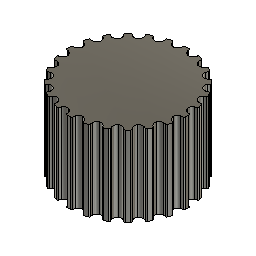
gear_24z (Autodesk Fusion 360 design; units mm, degrees)
Autodesk Fusion 360 part; units mm, degrees
sketch "Sketch1" plane through (0, 0, 0) normal (0, 0, 1) x (1, 0, 0) in component "gt2 pulley"
  circle A0 centre (0, 0) radius 7.6394 construction
  circle A1 centre (0, 0) radius 6.6354 construction
  line L0 (0, 0) -> (0, 7.6394) construction
  line L1 (0, 0) -> (0.9971, 7.5741) construction
  line L2 (0, 0) -> (1.4112, 7.508) construction
  circle A2 centre (0, 0) radius 7.3854 construction
  arc A3 (0.3646, 7.2357) -> (0.4075, 6.9675) centre (1.3643, 7.2583) ccw
  circle A4 centre (0, 0) radius 7.2354 construction
  arc A5 (0.219, 7.3822) -> (0, 7.3854) centre (0, 0) ccw
  arc A6 (0.3646, 7.2357) -> (0.219, 7.3822) centre (0.2146, 7.2323) ccw
  arc A7 (0.4075, 6.9675) -> (0.8661, 6.5787) centre (0.9385, 7.1289) ccw
  arc A8 (0, 7.3854) -> (-0.219, 7.3822) centre (0, 0) ccw
  arc A9 (-0.219, 7.3822) -> (-0.3646, 7.2357) centre (-0.2146, 7.2323) ccw
  arc A10 (-0.4075, 6.9675) -> (-0.3646, 7.2357) centre (-1.3643, 7.2583) ccw
  arc A11 (-0.866, 6.5787) -> (-0.4075, 6.9675) centre (-0.9385, 7.1289) ccw
  arc A12 (0.8661, 6.5787) -> (-0.8661, 6.5787) centre (0, 0) ccw
  point P0 (1.3643, 7.2583)
  point P1 (0, 7.3854)
  dimension "d18" = 15.2789
  dimension "d19" = 7.5
  dimension "d22" = 1.004
  dimension "d24" = 0.75
  dimension "d26" = 1
  dimension "d27" = 0.15
  dimension "d28" = 0.15
  dimension "d47" = 0.555
  dimension "d52" = 3.812
  constraint coincident A0.centre A1.centre
  constraint coincident A0 L0.end
  constraint vertical L0
  constraint coincident A0 L1.end
  constraint coincident A0 L2.end
  constraint concentric A1 A2
  constraint coincident A1 A7.end
  constraint coincident L1 A7.end
  constraint coincident A2 P0
  constraint coincident L2 P0
  constraint coincident P0 A3.centre
  constraint coincident A2 P1
  constraint coincident L0 P1
  constraint concentric A2 A4
  constraint coincident P1 A5.end
  constraint coincident A4 A6.centre
  constraint coincident A3.start A6.start
  constraint tangent A3 A6
  constraint tangent A3 A7
  constraint symmetric L0 A7.end A12.end
  constraint symmetric L0 A3.start A9.end
  constraint symmetric L0 A3.end A10.start
  constraint symmetric L0 A3 A10
  constraint symmetric L0 A5.start A8.end
  constraint symmetric L0 P1 A5.end
  constraint symmetric L0 A5 A8
  constraint symmetric L0 A6 A9
  constraint symmetric L0 A7 A11
  constraint coincident A1 A11.start
  constraint tangent A1 A7
  constraint coincident L1 A7.centre
  measures "d18" diameter of A0
  measures "d19" angle of L0 L1
  measures "d22" distance of A0 A1
  measures "d24" distance of A1 A2
  measures "d26" radius of A3
  measures "d27" distance of A2 A4
  measures "d28" radius of A6
  measures "d47" radius of A7
extrude "Extrude1" add sketch "Sketch1" along normal blind 10 makes body 1
pattern_circular "C-Pattern1" count 24 over 360 about axis through (0, 0, 1.75) along (0, 0, 1) of bodies 1 makes body 2 at (-2.3599, 6.2016, 6.6667) makes body 3 at (-3.8845, 5.3795, 6.6667) makes body 4 at (-4.1908, 5.1445, 3.3333) makes body 5 at (-5.3795, 3.8846, 3.3333) makes body 6 at (-6.2016, 2.3599, 3.3333) makes body 7 at (-6.6011, -0.6743, 6.6667) makes body 8 at (-6.2016, -2.3599, 6.6667) makes body 9 at (-6.0539, -2.7165, 3.3333) makes body 10 at (-5.1445, -4.1908, 3.3333) makes body 11 at (-3.2338, -5.7941, 6.6667) makes body 12 at (-2.3599, -6.2016, 3.3333) makes body 13 at (0.6743, -6.6011, 6.6667) makes body 14 at (2.3599, -6.2016, 6.6667) makes body 15 at (3.4009, -5.6976, 6.6667) makes body 16 at (4.1908, -5.1445, 3.3333) makes body 17 at (5.3795, -3.8846, 3.3333) makes body 18 at (6.2016, -2.3599, 3.3333) makes body 19 at (6.6011, 0.6743, 6.6667) makes body 20 at (6.2016, 2.3599, 6.6667) makes body 21 at (5.3795, 3.8845, 6.6667) makes body 22 at (5.1445, 4.1908, 3.3333) makes body 23 at (2.7165, 6.0539, 6.6667) makes body 24 at (1.0571, 6.5507, 6.6667)
sketch "Sketch2" plane through (0, 0, 10) normal (0, 0, 1) x (-1, 0, 0)
  arc A0 (-7.2357, 0.3646) -> (-7.3822, 0.219) centre (-7.2323, 0.2146) ccw
  arc A1 (-7.3822, 0.219) -> (-7.3822, -0.219) centre (0, 0) ccw
  arc A2 (-7.3822, -0.219) -> (-7.2357, -0.3646) centre (-7.2323, -0.2146) ccw
  arc A3 (-6.9675, -0.4075) -> (-7.2357, -0.3646) centre (-7.2583, -1.3643) ccw
  arc A4 (-6.5787, -0.866) -> (-6.9675, -0.4075) centre (-7.1289, -0.9385) ccw
  arc A5 (-6.5787, 0.8661) -> (-6.5787, -0.866) centre (0, 0) ccw
  arc A6 (-6.9675, 0.4075) -> (-6.5787, 0.8661) centre (-7.1289, 0.9385) ccw
  arc A7 (-7.2357, 0.3646) -> (-6.9675, 0.4075) centre (-7.2583, 1.3643) ccw
  circle A8 centre (0, 0) radius 6.6354
  constraint concentric A1 A8
extrude "Extrude2" add sketch "Sketch2" against normal blind 10 contours A5 A8 bodies 1 2 3 4 5 6 7 8 9 10 11 12 13 14 15 16 17 18 19 20 21 22 23 24
extrude "Extrude4" [suppressed] in component "gt2 pulley"
pattern_circular "C-Pattern7" [suppressed] in component "gt2 pulley"
extrude "Extrude3" [suppressed] in component "gt2 pulley"
pattern_circular "C-Pattern6" [suppressed] in component "gt2 pulley"
extrude "Extrude2'" [suppressed] in component "gt2 pulley"
pattern_circular "C-Pattern5" [suppressed] in component "gt2 pulley"
extrude "Extrude1'" [suppressed] in component "gt2 pulley"
pattern_circular "C-Pattern4" [suppressed] in component "gt2 pulley"
pattern_circular "C-Pattern3" [suppressed] in component "gt2 pulley"
pattern_circular "C-Pattern2" [suppressed] in component "gt2 pulley"
pattern_circular "C-Pattern1'" [suppressed] in component "gt2 pulley"
copy_body "Body->Comp1" [suppressed] in component "Component"
copy_body "Body->Comp2" [suppressed] in component "Component'"
copy_body "Body->Comp3" [suppressed] in component "Component''"
copy_body "Body->Comp4" [suppressed] in component "Component'''"
copy_body "Body->Comp5" [suppressed] in component "Component''''"
copy_body "Body->Comp6" [suppressed] in component "Component'''''"
copy_body "Body->Comp7" [suppressed] in component "Component''''''"
copy_body "Body->Comp8" [suppressed] in component "Component'''''''"
copy_body "Body->Comp9" [suppressed] in component "Component''''''''"
copy_body "Body->Comp10" [suppressed] in component "Component'''''''''"
copy_body "Body->Comp11" [suppressed] in component "Component''''''''''"
copy_body "Body->Comp12" [suppressed] in component "Component'''''''''''"
copy_body "Body->Comp13" [suppressed] in component "Component''''''''''''"
copy_body "Body->Comp14" [suppressed] in component "Component'''''''''''''"
copy_body "Body->Comp15" [suppressed] in component "Component''''''''''''''"
copy_body "Body->Comp16" [suppressed] in component "Component'''''''''''''''"
copy_body "Body->Comp17" [suppressed] in component "Component''''''''''''''''"
copy_body "Body->Comp18" [suppressed] in component "Component'''''''''''''''''"
copy_body "Body->Comp19" [suppressed] in component "Component''''''''''''''''''"
copy_body "Body->Comp20" [suppressed] in component "Component'''''''''''''''''''"
component "gt2 pulley" placed x (1, 0, 0) y (0, 1, 0) z (0, 0, 1) at (0, 0, 0)
equation "NumTeeth = 24" comment "min 20"
equation "ToothPitch = 2 mm"
equation "PullyDia = NumTeeth * ToothPitch / PI"
equation "ToothAng = ( ( 360 / NumTeeth ) * 1 deg )"
equation "TransOffsetAngle = ToothAng * 0.2"
equation "Sholulder_Radius = 0.15 mm"
equation "Root_Radius = 0.555 mm"
equation "TransRadius = 1 mm"
equation "ToolHeight = 0.75 mm"
equation "PLD = 0.254 mm"
equation "d18 = PullyDia"
equation "d19 = ToothAng / 2"
equation "d22 = PLD + ToolHeight"
equation "d24 = ToolHeight"
equation "d26 = TransRadius"
equation "d27 = Sholulder_Radius"
equation "d31 = NumTeeth"
equation "d33 = NumTeeth"
equation "d35 = NumTeeth"
equation "d37 = NumTeeth"
equation "d41 = NumTeeth"
equation "d45 = NumTeeth"
equation "d47 = Root_Radius"
equation "d50 = NumTeeth"
